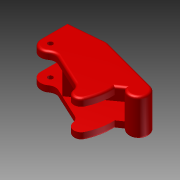
# Autodesk Inventor part: 03
Saved by Autodesk Inventor 2012 (Build 160160000, 160)
## iProperties
Created: 2014-01-27
Part Number: 03
Material: Default
Document SubType Name: Modeling
Designer: Michał
Density: 1 g/cm^3
Author: Michał
Autodesk Inventor part; units mm, degrees
ref_plane "YZ Plane" through (0, 0, 0) normal (1, 0, 0) x (0, 1, 0)
ref_plane "XZ Plane" through (0, 0, 0) normal (0, 1, 0) x (-1, 0, 0)
ref_plane "XY Plane" through (0, 0, 0) normal (0, 0, 1) x (1, 0, 0)
sketch "Sketch1" plane through (0, 0, 0) normal (0, 0, 1) x (1, 0, 0)
  line L0 (0, 0) -> (0, 11)
  line L1 (0, 11) -> (14.9429, 12.3073)
  line L2 (14.9429, 12.3073) -> (39.0911, 5.8369)
  arc A0 (34.7792, -0.3211) -> (39.0911, 5.8369) centre (38.0558, 1.9732) ccw
  line L3 (34.7792, -0.3211) -> (32.3217, -2.0419)
  line L4 (38.0558, 1.9732) -> (45.0558, 1.9732) construction
  arc A1 (0, 0) -> (7.6252, -1.6905) centre (4, 0) ccw
  line L5 (7.6252, -1.6905) -> (24.8451, -9.7202)
  line L6 (4, 0) -> (27, 0) construction
  arc A2 (24.8451, -9.7202) -> (30.2845, -12.2526) centre (27.564, -10.9881) ccw
  arc A3 (30.2845, -12.2526) -> (32.3217, -2.0419) centre (10.273, -2.9513) ccw
  circle A4 centre (4, 0) radius 1
  dimension "d0" = 11
  dimension "d1" = 15
  dimension "d2" = 95
  dimension "d3" = 25
  dimension "d4" = 160
  dimension "d6" = 7
  dimension "d7" = 145
  dimension "d8" = 23
  dimension "d9" = 25
  dimension "d10" = 3
  dimension "d11" = 2
  constraints: 14 end point, 8 point on circle, 5 centre point, 2 horizontal, 2 point on line, 2 tangent, 1 coincident, 1 vertical
  measures "d0" distance of L0.start L0.end
  measures "d1" distance of L0.end L1.end
  measures "d2" angle of L0 L1
  measures "d3" distance of L1.end L2.end
  measures "d4" angle of L1 L2
  measures "d6" distance of L4.start L3.end
  measures "d7" angle of L3 L4
  measures "d8" distance of L6.start L5.end
  measures "d9" angle of L5 L6
  measures "d10" distance of L5.end A2.centre
  measures "d11" diameter of A4
extrude "Extrusion1" add sketch "Sketch1" along normal blind 3
sketch "Sketch2" plane through (0, 0, 0) normal (0, 0, -1) x (-1, 0, 0)
  line L0 (0, 11) -> (0, 0) projected
  line L1 (-14.9429, 12.3073) -> (0, 11) projected
  line L2 (-39.0911, 5.8369) -> (-14.9429, 12.3073) projected
  arc A0 (-39.0911, 5.8369) -> (-34.7792, -0.3211) centre (-38.0558, 1.9732) ccw projected
  line L3 (-7.6252, -1.6905) -> (-24.8451, -9.7202) projected
  arc A1 (-7.6252, -1.6905) -> (0, 0) centre (-4, 0) ccw projected
  line L4 (-28.1718, 6.8009) -> (-35.3153, 4.8868)
  arc A2 (-39.0911, 5.8369) -> (-35.3153, 4.8868) centre (-38.0558, 1.9732) ccw
  line L5 (-4, 0) -> (-13.0631, -4.2262)
  line L6 (-13.0631, -4.2262) -> (-28.1718, 6.8009)
  line L7 (-13.0631, -4.2262) -> (-12.4735, -3.4184)
  line L8 (-27.017, 7.1961) -> (-14.6534, 10.5089)
  line L9 (-14.6534, 10.5089) -> (0, 9.2269)
  line L10 (-27.017, 7.1961) -> (-12.4735, -3.4184)
  line L11 (0, 9.2269) -> (0, 11)
  line L12 (0, 11) -> (-14.9429, 12.3073)
  line L13 (-14.9429, 12.3073) -> (-39.0911, 5.8369)
  dimension "d15" = 11
  dimension "d16" = 10
  dimension "d17" = 1
  constraints: 20 end point, 4 parallel, 3 point on circle, 3 point on line, 2 collinear, 2 perpendicular, 2 tangent, 1 centre point, 1 coincident
  measures "d15" distance of L4.start A0.centre
  measures "d16" distance of L5.start L5.end
  measures "d17" distance of L5.end L7.end
extrude "Extrusion2" add sketch "Sketch2" along normal blind 4.5 contours L0 L9 L8 L10 L7 L6 L4 A2 A0 L2 L1
fillet "Fillet2" radius 3.5 3 edges at (24.8451, -9.7202, 1.5) (7.6252, -1.6905, 1.5) (14.9429, 12.3073, -0.75)
fillet "Fillet1" radius 1 9 edges at (41.3324, -0.3211, 3) (27.3151, 8.9922, 3) (33.5505, -1.1815, 3) (27.1115, -13.9538, 3) (31.9139, -7.2691, 3) (16.3059, -5.7383, 3) (0, 5.5, 3) (2.2209, -3.5826, 3) (7.1641, 11.6268, 3)
sketch "Sketch3" plane through (14.3281, 12.2535, 2) normal (-0.0871557, 0.9961947, 0) x (0.9961947, 0.0871557, 0)
  line L0 (0, 6.5) -> (-14.3829, 6.5) projected
  line L1 (-14.3829, 0) -> (-14.3829, 6.5) projected
  line L2 (-14.5374, 2) -> (-14.5374, 6.5) projected
  arc A0 (-14.3829, 2) -> (-11.8008, 6.5) centre (-17.0132, 6.5) ccw
  line L3 (-11.8008, 6.5) -> (-14.3829, 6.5)
  line L4 (-14.3829, 2) -> (-14.3829, 6.5)
  point P0 (-15.3416, 2)
  constraints: 4 end point, 2 collinear, 2 point on circle, 2 point on line, 1 centre point
extrude "Extrusion3" cut sketch "Sketch3" against normal up to surface (1.7664 mm away)
sketch "Sketch4" plane through (0, 9.2269, -4.5) normal (0.0871557, -0.9961947, 0) x (0.9961947, 0.0871557, 0)
  line L0 (0.1545, 0) -> (0.1545, 4.5) projected
  line L1 (0, 4.5) -> (0.1545, 4.5) projected
  line L2 (0, 4.5) -> (0, 0) projected
  line L3 (0, 0) -> (0.1545, 0) projected
  point P0 (-0.8042, 4.5)
extrude "Extrusion4" cut sketch "Sketch4" against normal up to surface (1.7664 mm away)
mirror "Mirror1" about plane through (21.7965, 5.9413, -4.5) normal (0, 0, -1) of "Extrusion1", "Extrusion2", "Fillet2", "Fillet1", "Extrusion3", "Extrusion4"
body "Solid1"
